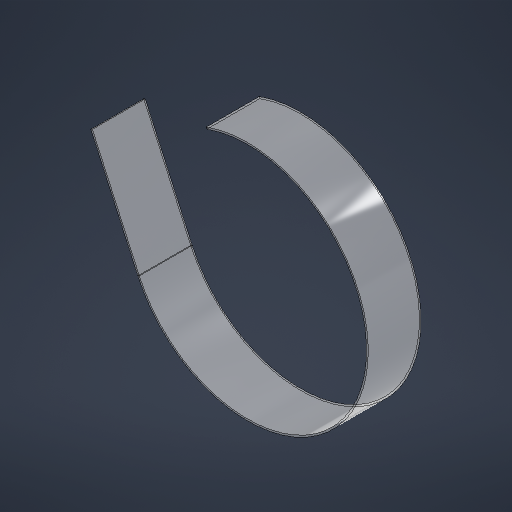
# Autodesk Inventor part: PLATE,WALL
Saved by Autodesk Inventor 2026 (Build 300175000, 175)
## iProperties
Created: 2026-02-06
Part Number: PLATE,WALL
Material: Polycarbonate, Clear
Document SubType Name: Sheet Metal
Designer: littl
Density: 1.2 g/cm^3
Sheet Metal Rule: Default
Appearance: Polycarbonate - Clear
Author: littl
Autodesk Inventor part; units mm, degrees
ref_plane "YZ Plane" through (0, 0, 0) normal (1, 0, 0) x (0, 1, 0)
ref_plane "XZ Plane" through (0, 0, 0) normal (0, 1, 0) x (-1, 0, 0)
ref_plane "XY Plane" through (0, 0, 0) normal (0, 0, 1) x (1, 0, 0)
sketch "Sketch2" plane through (0, 0, 0) normal (0, 0, 1) x (1, 0, 0)
  line L0 (349.25, -349.25) -> (-349.25, -349.25) construction
  line L1 (-349.25, -349.25) -> (-349.25, 349.25) construction
  line L2 (-349.25, 349.25) -> (349.25, 349.25) construction
  line L3 (349.25, 349.25) -> (349.25, -349.25) construction
  line L4 (349.25, -349.25) -> (-349.25, 349.25) construction
  line L5 (-349.25, -349.25) -> (349.25, 349.25) construction
  circle A0 centre (-158.75, 158.75) radius 190.5 construction
  circle A1 centre (274.0629, -88.8699) radius 75.057 construction
  circle A2 centre (174.0677, 61.4014) radius 75.057 construction
  circle A3 centre (0.2511, 12.7367) radius 75.057 construction
  circle A4 centre (-7.1783, -167.611) radius 75.057 construction
  circle A5 centre (162.0466, -230.4073) radius 75.057 construction
  arc A6 (-85.9497, -180.3996) -> (-87.5155, -177.0226) centre (120.65, -82.55) ccw construction
  circle A7 centre (-158.75, 158.75) radius 79.375 construction
  line L6 (-87.014, 192.7256) -> (-63.9106, 143.9451) construction
  line L7 (-230.486, 124.7744) -> (-87.014, 192.7256) construction
  circle A8 centre (-20.4963, 117.3988) radius 38.1 construction
  line L8 (-264.4615, 196.5104) -> (-120.9896, 264.4615) construction
  line L9 (-264.4615, 196.5104) -> (-230.486, 124.7744) construction
  line L10 (-120.9896, 264.4615) -> (-87.014, 192.7256) construction
  circle A9 centre (-81.3983, -14.6583) radius 75.057 construction
  line L11 (42.4642, 132.2637) -> (120.65, -82.55) construction
  line L12 (-161.9258, 76.4446) -> (-93.0592, 109.0612) construction
  line L13 (-93.0592, 109.0612) -> (-75.3919, 71.7584) construction
  line L14 (-75.3919, 71.7584) -> (-144.2585, 39.1419) construction
  line L15 (-144.2585, 39.1419) -> (-161.9258, 76.4446) construction
  line L16 (-161.9258, 76.4446) -> (-75.3919, 71.7584) construction
  line L17 (-93.0592, 109.0612) -> (-144.2585, 39.1419) construction
  line L18 (-127.4925, 92.7529) -> (-124.7744, 87.014) construction
  line L19 (-124.7744, 87.014) -> (-118.6588, 74.1015) construction
  line L20 (-85.9497, -180.3996) -> (-170.209, -2.4943) construction
  line L21 (-170.209, -2.4943) -> (-230.486, 124.7744) construction
  line L22 (-503.9407, 0) -> (578.8945, 0)
  line L23 (-87.5155, -177.0226) -> (-177.7325, 21.7659)
  arc A10 (-87.5155, -177.0226) -> (42.4642, 132.2637) centre (120.65, -82.55) ccw
  point P0 (0, 0)
  point P1 (0, 0)
  dimension "d15" = 698.5
  dimension "d16" = 698.5
  dimension "d17" = 381
  dimension "d18" = 190.5
  dimension "d19" = 190.5
  dimension "d20" = 150.114
  dimension "d21" = 360
  dimension "d22" = 228.6
  dimension "d23" = 158.75
  dimension "d24" = 76.2
  dimension "d25" = 266.7
  dimension "d26" = 228.6
  dimension "d27" = 244.7484
  dimension "d28" = 231.8512
  dimension "d29" = 133.35
  dimension "d32" = 41.275
  dimension "d33" = 76.2
  dimension "d34" = 6.35
  dimension "d35" = 196.85
  dimension "d47" = 70
  dimension "d48" = 25.4
  dimension "d50" = 3.175
  measures "d15" distance of L1.end L2.end
  measures "d16" distance of L0.end L1.end
  measures "d17" diameter of A0
  measures "d18" distance from line of L1 A0.centre
  measures "d19" distance from line of L2 A0.centre
  measures "d20" diameter of A1
  measures "d22" radius of A6
  measures "d23" diameter of A7
  measures "d24" diameter of A8
  measures "d25" distance from line of L0 L11.end
  measures "d26" distance from line of L3 point (120.65, -82.55)
  measures "d27" distance of point (120.65, -82.55) A8.centre
  measures "d28" distance from line of A8.centre L2
  measures "d29" distance of L8.end L6.end
  measures "d32" distance of L14.end L12.start
  measures "d33" distance of L12.start L12.end
  measures "d34" distance of L18.start L18.end
  measures "d35" distance of L20.start L20.end
  measures "d47" angle of L22 L11
  measures "d48" distance of L20.end L23.end
  measures "d50" distance from line of L20.end L23
contour flange "Contour Flange2" sketch "Sketch2" thickness 3.175 bend radius 3.175 width 101.6 along (0, 0, 1) mid plane no both sides no wall seen from (-132.624, -77.6283, 0) lies toward (-0.9106104, -0.4132658, 0) curves L23 A10
bend "Bend2"
corner "Corner2"
equation "\"d19\" = d18"
equation "\"d36\" = Thickness"
equation "\"d37\" = BendReliefWidth"
equation "\"d38\" = BendReliefDepth"
equation "\"d39\" = MinimumRemnant"
equation "\"d40\" = TransitionRadius"
equation "\"d42\" = BendRadius"
equation "\"d44\" = CornerReliefSize"
equation "\"d45\" = GapSize"
equation "\"d46\" = JacobiRadiusSize"
equation "\"BendRadius\" = Thickness"
equation "\"BendReliefWidth\" = Thickness"
equation "\"BendReliefDepth\" = 0.5 * Thickness"
equation "\"CornerReliefSize\" = 4 * Thickness"
equation "\"MinimumRemnant\" = 2 * Thickness"
equation "\"TransitionRadius\" = BendRadius"
equation "\"JacobiRadiusSize\" = BendRadius"
equation "\"GapSize\" = Thickness"
equation "\"Thickness\" = 3.175"
body "Solid2"
